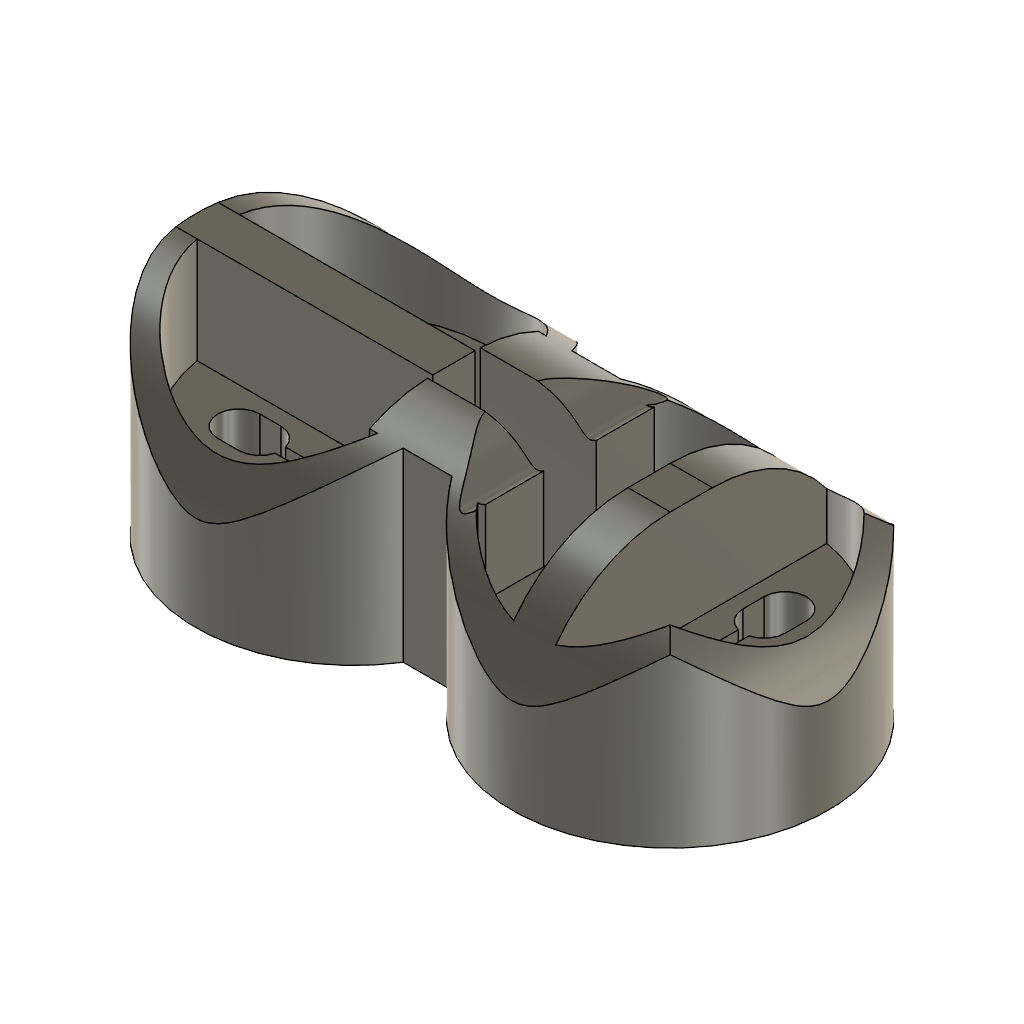
Sensor case Top V1 (Autodesk Fusion 360 design; units mm, degrees)
part number: 2026-09-03-18-15-27-787
Autodesk Fusion 360 part; units mm, degrees
note: some values were not read from the file. Set by a fixed rule: which sketch regions a step uses.
sketch "Sketch1" plane through (0, 0, 0) normal (0, 0, 1) x (1, 0, 0)
  line L0 (1.1557, 4) -> (-1.1557, 4)
  line L1 (1.1557, -4) -> (-1.1557, -4)
  arc A0 (-1.1557, 4) -> (-1.1557, -4) centre (-7.5, 0) ccw
  arc A1 (1.1557, -4) -> (1.1557, 4) centre (7.5, 0) ccw
  line L2 (2.75, 0) -> (-2.75, 0)
  line L3 (0, -1.25) -> (0, 1.25)
  line L4 (-2.75, -1.25) -> (-2.75, 1.25)
  line L5 (2.75, -1.25) -> (2.75, 1.25)
  line L6 (-2.75, 1.25) -> (2.75, 1.25)
  line L7 (2.75, 1.25) -> (2.75, -1.25)
  line L8 (2.75, -1.25) -> (-2.75, -1.25)
  line L9 (-2.75, -1.25) -> (-2.75, 1.25)
  point P0 (0, 4)
  point P1 (0, -4)
  dimension "d1" = 15
  dimension "d2" = 5.5
  dimension "d3" = 2.5
  dimension "d4" = 2.5
  dimension "d5" = 2.5
  constraint coincident origin A0
  constraint coincident origin A1
  constraint midpoint L0 P0
  constraint horizontal L0
  constraint midpoint L1 P1
  constraint horizontal L1
  constraint midpoint L2 origin
  constraint horizontal L2
  constraint midpoint L3 origin
  constraint perpendicular L2 L3
  constraint horizontal L6
  constraint vertical L7
  constraint horizontal L8
  constraint vertical L9
  measures "d1" diameter of A1
  measures "d2" distance of L2.start L2.end
  measures "d3" distance of L3.start L3.end
  measures "d4" distance of L4.start L4.end
  measures "d5" distance of L5.start L5.end
extrude "Extrude1" add sketch "Sketch1" along normal blind 4.5
sketch "Sketch2" plane through (0, 0, 4.5) normal (0, 0, 1) x (-1, 0, 0)
  line L0 (-2.75, 1.25) -> (2.75, 1.25)
  line L1 (2.75, 1.25) -> (2.75, -1.25)
  line L2 (2.75, -1.25) -> (-2.75, -1.25)
  line L3 (-2.75, -1.25) -> (-2.75, 1.25)
  arc A0 (-1.1557, 4) -> (-1.1557, -4) centre (-7.5, 0) ccw
  line L4 (-1.1557, -4) -> (1.1557, -4)
  arc A1 (1.1557, -4) -> (1.1557, 4) centre (7.5, 0) ccw
  line L5 (1.1557, 4) -> (-1.1557, 4)
  line L6 (7.5, 1) -> (7.5, -1)
  line L7 (7.5, -1) -> (7.5, -2.7)
  line L8 (9.25, -2.7) -> (5.75, -2.7)
  line L9 (9.2781, -3.6996) -> (10.2496, -3.7)
  line L10 (9.25, -1.7) -> (10.25, -1.7)
  line L11 (4.75, -3.7) -> (5.75, -3.7)
  line L12 (4.75, -1.7) -> (5.75, -1.7)
  arc A2 (9.25, -1.7) -> (9.2781, -3.6996) centre (9.25, -2.7) ccw
  arc A3 (10.2496, -3.7) -> (10.25, -1.7) centre (10.25, -2.7) ccw
  arc A4 (5.7496, -3.7) -> (5.75, -1.7) centre (5.75, -2.7) ccw
  arc A5 (4.75, -1.7) -> (4.7504, -3.7) centre (4.75, -2.7) ccw
  line L13 (10.25, 1.7) -> (9.25, 1.7)
  arc A6 (9.2504, 3.7) -> (9.25, 1.7) centre (9.25, 2.7) ccw
  line L14 (10.25, 3.7) -> (9.25, 3.7)
  arc A7 (10.25, 1.7) -> (10.2496, 3.7) centre (10.25, 2.7) ccw
  arc A8 (5.75, 1.7) -> (5.7219, 3.6996) centre (5.75, 2.7) ccw
  line L15 (5.7219, 3.6996) -> (4.7504, 3.7)
  line L16 (5.75, 1.7) -> (4.75, 1.7)
  arc A9 (4.7504, 3.7) -> (4.75, 1.7) centre (4.75, 2.7) ccw
  line L17 (5.75, 2.7) -> (9.25, 2.7)
  line L18 (7.5, 1) -> (7.5, 2.7)
  line L19 (7.5, -1) -> (7.5, 1)
  line L20 (-6.5, 0) -> (-8.5, 0)
  line L21 (-8.5, 0) -> (-10.2, 0)
  line L22 (-10.2, -1.75) -> (-10.2, 1.75)
  arc A10 (-9.2, -1.75) -> (-11.1996, -1.7781) centre (-10.2, -1.75) ccw
  line L23 (-9.2, -1.75) -> (-9.2, -2.75)
  arc A11 (-11.2, -2.7496) -> (-9.2, -2.75) centre (-10.2, -2.75) ccw
  line L24 (-11.1996, -1.7781) -> (-11.2, -2.7496)
  line L25 (-11.2, 2.75) -> (-11.2, 1.75)
  arc A12 (-11.2, 1.7504) -> (-9.2, 1.75) centre (-10.2, 1.75) ccw
  arc A13 (-9.2, 2.75) -> (-11.2, 2.7496) centre (-10.2, 2.75) ccw
  line L26 (-9.2, 2.75) -> (-9.2, 1.75)
  line L27 (-6.5, 0) -> (-4.8, 0)
  line L28 (-4.8, 1.75) -> (-4.8, -1.75)
  arc A14 (-5.8, 1.75) -> (-3.8004, 1.7781) centre (-4.8, 1.75) ccw
  line L29 (-5.8, 1.75) -> (-5.8, 2.75)
  arc A15 (-3.8, 2.7496) -> (-5.8, 2.75) centre (-4.8, 2.75) ccw
  line L30 (-3.8004, 1.7781) -> (-3.8, 2.7496)
  line L31 (-3.8, -2.75) -> (-3.8, -1.75)
  arc A16 (-5.8, -2.75) -> (-3.8, -2.7496) centre (-4.8, -2.75) ccw
  line L32 (-5.8, -2.75) -> (-5.8, -1.75)
  arc A17 (-3.8, -1.7504) -> (-5.8, -1.75) centre (-4.8, -1.75) ccw
  point P0 (7.5, 0)
  dimension "d8" = 2
  dimension "d9" = 1.7
  dimension "d10" = 3.5
  dimension "d11" = 2
  dimension "d12" = 2
  dimension "d13" = 2
  dimension "d14" = 2
  dimension "d15" = 2
  dimension "d16" = 1.7
  dimension "d17" = 3.5
  dimension "d18" = 2
  dimension "d19" = 2
  dimension "d20" = 2
  dimension "d21" = 2
  dimension "d22" = 2
  dimension "d23" = 1.7
  dimension "d24" = 3.5
  dimension "d25" = 2
  dimension "d26" = 2
  dimension "d27" = 2
  dimension "d28" = 2
  dimension "d29" = 1.7
  dimension "d30" = 3.5
  dimension "d31" = 2
  dimension "d32" = 2
  dimension "d33" = 2
  dimension "d34" = 2
  constraint midpoint L6 P0
  constraint coincident P0 A1.centre
  constraint vertical L6
  constraint parallel L6 L7
  constraint midpoint L7.end L8
  constraint perpendicular L7 L8
  constraint coincident L8.start A2.centre
  constraint coincident L8.end A4.centre
  constraint coincident L9.end A3
  constraint tangent L9 A3
  constraint tangent L10 A3
  constraint parallel L8 L10
  constraint coincident L9 A3.start
  constraint coincident L11 A5.end
  constraint coincident L11 A4.start
  constraint parallel L18 L19
  constraint midpoint L18.end L17
  constraint perpendicular L17 L18
  constraint coincident A8.centre L17.start
  constraint coincident A6.centre L17.end
  constraint coincident L15.end A9
  constraint tangent L15 A9
  constraint tangent L16 A9
  constraint parallel L16 L17
  constraint coincident A9.start L15
  constraint coincident A7.end L14
  constraint coincident A6.start L14
  constraint parallel L20 L21
  constraint midpoint L21.end L22
  constraint perpendicular L21 L22
  constraint coincident L22.start A10.centre
  constraint coincident L22.end A12.centre
  constraint coincident L24.end A11
  constraint tangent A11 L24
  constraint tangent L23 A11
  constraint parallel L22 L23
  constraint coincident A11.start L24
  constraint coincident A13.end L25
  constraint coincident A12.start L25
  constraint midpoint L27.end L28
  constraint perpendicular L27 L28
  constraint coincident L28.start A14.centre
  constraint coincident L28.end A17.centre
  constraint coincident L30.end A15
  constraint tangent A15 L30
  constraint tangent L29 A15
  constraint parallel L28 L29
  constraint coincident A15.start L30
  constraint coincident A16.end L31
  constraint coincident A17.start L31
  measures "d8" distance of L6.start L6.end
  measures "d9" distance of L6.end L7.end
  measures "d10" distance of L8.start L8.end
  measures "d11" diameter of A2
  measures "d12" diameter of A4
  measures "d13" diameter of A3
  measures "d14" diameter of A5
  measures "d15" distance of L6.end L6.start
  measures "d16" distance of L6.start L18.end
  measures "d17" distance of A8.centre A6.centre
  measures "d18" diameter of A8
  measures "d19" diameter of A6
  measures "d20" diameter of A9
  measures "d21" diameter of A7
  measures "d22" distance of L20.start L20.end
  measures "d23" distance of L20.end L21.end
  measures "d24" distance of L22.start L22.end
  measures "d25" diameter of A10
  measures "d26" diameter of A12
  measures "d27" diameter of A11
  measures "d28" diameter of A13
  measures "d29" distance of L27.end L20.start
  measures "d30" distance of L28.end L28.start
  measures "d31" diameter of A14
  measures "d32" diameter of A17
  measures "d33" diameter of A15
  measures "d34" diameter of A16
extrude "Extrude2" cut sketch "Sketch2" against normal blind 5 contours L9 L10 A2 A3 | L11 L12 A4 A5 | L13 A6 L14 A7 | A8 L15 L16 A9 | A10 L23 A11 L24 | L25 A12 A13 L26 | A14 L29 A15 L30 | L31 A16 L32 A17
sketch "Sketch3" plane through (0, 0, 4.5) normal (0, 0, 1) x (-1, 0, 0)
  arc A0 (-1.1557, 4) -> (-1.1557, -4) centre (-7.5, 0) ccw
  line L0 (-1.1557, -4) -> (1.1557, -4)
  arc A1 (1.1557, -4) -> (1.1557, 4) centre (7.5, 0) ccw
  line L1 (1.1557, 4) -> (-1.1557, 4)
  line L2 (-2.75, 1.25) -> (2.75, 1.25)
  line L3 (2.75, 1.25) -> (2.75, -1.25)
  line L4 (2.75, -1.25) -> (-2.75, -1.25)
  line L5 (-2.75, -1.25) -> (-2.75, 1.25)
  line L6 (-3.8, 2.7496) -> (-3.8004, 1.7781)
  arc A2 (-5.8, 1.75) -> (-3.8004, 1.7781) centre (-4.8, 1.75) ccw
  line L7 (-5.8, 1.75) -> (-5.8, 2.75)
  arc A3 (-3.8, 2.7496) -> (-5.8, 2.75) centre (-4.8, 2.75) ccw
  line L8 (9.25, 3.7) -> (10.2496, 3.7)
  arc A4 (10.25, 1.7) -> (10.2496, 3.7) centre (10.25, 2.7) ccw
  line L9 (10.25, 1.7) -> (9.25, 1.7)
  arc A5 (9.25, 3.7) -> (9.25, 1.7) centre (9.25, 2.7) ccw
  line L10 (10.2496, -3.7) -> (9.2781, -3.6996)
  arc A6 (9.25, -1.7) -> (9.2781, -3.6996) centre (9.25, -2.7) ccw
  line L11 (9.25, -1.7) -> (10.25, -1.7)
  arc A7 (10.2496, -3.7) -> (10.25, -1.7) centre (10.25, -2.7) ccw
  line L12 (-3.8, -1.7504) -> (-3.8, -2.7496)
  arc A8 (-5.8, -2.75) -> (-3.8, -2.7496) centre (-4.8, -2.75) ccw
  line L13 (-5.8, -2.75) -> (-5.8, -1.75)
  arc A9 (-3.8, -1.7504) -> (-5.8, -1.75) centre (-4.8, -1.75) ccw
  arc A10 (-11.2, 1.7504) -> (-9.2, 1.75) centre (-10.2, 1.75) ccw
  line L14 (-11.2, 1.7504) -> (-11.2, 2.7496)
  arc A11 (-9.2, 2.75) -> (-11.2, 2.7496) centre (-10.2, 2.75) ccw
  line L15 (-9.2, 2.75) -> (-9.2, 1.75)
  line L16 (4.7504, 3.7) -> (5.7219, 3.6996)
  arc A12 (5.75, 1.7) -> (5.7219, 3.6996) centre (5.75, 2.7) ccw
  line L17 (5.75, 1.7) -> (4.75, 1.7)
  arc A13 (4.7504, 3.7) -> (4.75, 1.7) centre (4.75, 2.7) ccw
  line L18 (5.7496, -3.7) -> (4.7504, -3.7)
  arc A14 (4.75, -1.7) -> (4.7504, -3.7) centre (4.75, -2.7) ccw
  line L19 (4.75, -1.7) -> (5.75, -1.7)
  arc A15 (5.7496, -3.7) -> (5.75, -1.7) centre (5.75, -2.7) ccw
  line L20 (-11.2, -2.7496) -> (-11.1996, -1.7781)
  arc A16 (-9.2, -1.75) -> (-11.1996, -1.7781) centre (-10.2, -1.75) ccw
  line L21 (-9.2, -1.75) -> (-9.2, -2.75)
  arc A17 (-11.2, -2.7496) -> (-9.2, -2.75) centre (-10.2, -2.75) ccw
  line L22 (7.5, 2.7) -> (7.5, -2.7)
  line L23 (6.7182, -2.45) -> (8.2818, -2.45)
  line L24 (8.2818, -2.45) -> (8.2818, -2.95)
  line L25 (8.2818, -2.95) -> (6.7182, -2.95)
  line L26 (6.7182, -2.95) -> (6.7182, -2.45)
  line L27 (6.7182, -2.45) -> (8.2818, -2.95) construction
  line L28 (8.2818, -2.45) -> (6.7182, -2.95) construction
  line L29 (6.7182, -2.45) -> (8.2818, -2.45)
  line L30 (8.2818, -2.95) -> (6.7182, -2.95)
  line L31 (8.2818, -2.45) -> (8.2818, -2.95)
  line L32 (6.7182, -2.95) -> (6.7182, -2.45)
  line L33 (6.7182, 2.95) -> (8.2818, 2.95)
  line L34 (8.2818, 2.45) -> (6.7182, 2.45)
  line L35 (8.2818, 2.95) -> (8.2818, 2.45)
  line L36 (6.7182, 2.45) -> (6.7182, 2.95)
  line L37 (-10.2, 0) -> (-4.8, 0)
  line L38 (-5.05, -0.7818) -> (-5.05, 0.7818)
  line L39 (-4.55, 0.7818) -> (-4.55, -0.7818)
  line L40 (-5.05, 0.7818) -> (-4.55, 0.7818)
  line L41 (-4.55, -0.7818) -> (-5.05, -0.7818)
  line L42 (-10.45, -0.7818) -> (-10.45, 0.7818)
  line L43 (-9.95, 0.7818) -> (-9.95, -0.7818)
  line L44 (-10.45, 0.7818) -> (-9.95, 0.7818)
  line L45 (-9.95, -0.7818) -> (-10.45, -0.7818)
  point P0 (7.5, 0)
  point P1 (7.5, -2.7)
  point P2 (-7.5, 0)
  dimension "d37" = 5.4
  dimension "d38" = 0.5
  dimension "d39" = 0.5
  dimension "d40" = 0.5
  dimension "d41" = 5.4
  dimension "d42" = 0.5
  dimension "d43" = 0.5
  constraint midpoint L22 P0
  constraint coincident P0 A1.centre
  constraint vertical L22
  constraint horizontal L23
  constraint perpendicular L23 L24
  constraint parallel L23 L25
  constraint parallel L24 L26
  constraint coincident L27 P1
  constraint coincident L28 P1
  constraint coincident A15 L23.start
  constraint coincident P1 L22.end
  constraint horizontal L29
  constraint perpendicular L29 L31
  constraint parallel L29 L30
  constraint parallel L31 L32
  constraint horizontal L33
  constraint perpendicular L33 L35
  constraint parallel L33 L34
  constraint parallel L35 L36
  constraint midpoint L37 P2
  constraint coincident P2 A0.centre
  constraint horizontal L37
  constraint perpendicular L38 L40
  constraint parallel L38 L39
  constraint parallel L40 L41
  constraint perpendicular L42 L44
  constraint parallel L42 L43
  constraint parallel L44 L45
  measures "d37" distance of L22.start P1
  measures "d38" distance of L23.end L24.end
  measures "d39" distance of L23.end L24.end
  measures "d40" distance of L33.end L34.start
  measures "d41" distance of L37.start L37.end
  measures "d42" distance of L38.end L39.start
  measures "d43" distance of L42.end L43.start
extrude "Extrude3" cut sketch "Sketch3" against normal blind 3 contours A2 A9 L38 L39 | A5 A12 L33 L34 | A6 A15 L23 L25 L29 L30 | A10 A16 L42 L43
sketch "Sketch4" plane through (0, 0, 4.5) normal (0, 0, 1) x (-1, 0, 0)
  line L0 (-10.45, -0.7818) -> (-10.45, 0.7818)
  arc A0 (-11.2, 1.7504) -> (-10.45, 0.7818) centre (-10.2, 1.75) ccw
  line L1 (-11.2, 1.7504) -> (-11.2, 2.7496)
  arc A1 (-9.2, 2.75) -> (-11.2, 2.7496) centre (-10.2, 2.75) ccw
  line L2 (-9.2, 2.75) -> (-9.2, 1.75)
  arc A2 (-9.95, 0.7818) -> (-9.2, 1.75) centre (-10.2, 1.75) ccw
  line L3 (-9.95, 0.7818) -> (-9.95, -0.7818)
  arc A3 (-9.2, -1.75) -> (-9.95, -0.7818) centre (-10.2, -1.75) ccw
  line L4 (-9.2, -1.75) -> (-9.2, -2.75)
  arc A4 (-11.2, -2.7496) -> (-9.2, -2.75) centre (-10.2, -2.75) ccw
  line L5 (-11.2, -2.7496) -> (-11.1996, -1.7781)
  arc A5 (-10.45, -0.7818) -> (-11.1996, -1.7781) centre (-10.2, -1.75) ccw
  line L6 (6.7182, -2.45) -> (8.2818, -2.45)
  arc A6 (9.25, -1.7) -> (8.2818, -2.45) centre (9.25, -2.7) ccw
  line L7 (9.25, -1.7) -> (10.25, -1.7)
  arc A7 (10.2496, -3.7) -> (10.25, -1.7) centre (10.25, -2.7) ccw
  line L8 (10.2496, -3.7) -> (9.2781, -3.6996)
  arc A8 (8.2818, -2.95) -> (9.2781, -3.6996) centre (9.25, -2.7) ccw
  line L9 (8.2818, -2.95) -> (6.7182, -2.95)
  arc A9 (5.7496, -3.7) -> (6.7182, -2.95) centre (5.75, -2.7) ccw
  line L10 (5.7496, -3.7) -> (4.7504, -3.7)
  arc A10 (4.75, -1.7) -> (4.7504, -3.7) centre (4.75, -2.7) ccw
  line L11 (4.75, -1.7) -> (5.75, -1.7)
  arc A11 (6.7182, -2.45) -> (5.75, -1.7) centre (5.75, -2.7) ccw
  line L12 (6.7182, 2.95) -> (8.2818, 2.95)
  arc A12 (9.25, 3.7) -> (8.2818, 2.95) centre (9.25, 2.7) ccw
  line L13 (9.25, 3.7) -> (10.2496, 3.7)
  arc A13 (10.25, 1.7) -> (10.2496, 3.7) centre (10.25, 2.7) ccw
  line L14 (10.25, 1.7) -> (9.25, 1.7)
  arc A14 (8.2818, 2.45) -> (9.25, 1.7) centre (9.25, 2.7) ccw
  line L15 (8.2818, 2.45) -> (6.7182, 2.45)
  arc A15 (5.75, 1.7) -> (6.7182, 2.45) centre (5.75, 2.7) ccw
  line L16 (5.75, 1.7) -> (4.75, 1.7)
  arc A16 (4.7504, 3.7) -> (4.75, 1.7) centre (4.75, 2.7) ccw
  line L17 (4.7504, 3.7) -> (5.7219, 3.6996)
  arc A17 (6.7182, 2.95) -> (5.7219, 3.6996) centre (5.75, 2.7) ccw
  line L18 (-5.05, -0.7818) -> (-5.05, 0.7818)
  arc A18 (-5.8, 1.75) -> (-5.05, 0.7818) centre (-4.8, 1.75) ccw
  line L19 (-5.8, 1.75) -> (-5.8, 2.75)
  arc A19 (-3.8, 2.7496) -> (-5.8, 2.75) centre (-4.8, 2.75) ccw
  line L20 (-3.8, 2.7496) -> (-3.8004, 1.7781)
  arc A20 (-4.55, 0.7818) -> (-3.8004, 1.7781) centre (-4.8, 1.75) ccw
  line L21 (-4.55, 0.7818) -> (-4.55, -0.7818)
  arc A21 (-3.8, -1.7504) -> (-4.55, -0.7818) centre (-4.8, -1.75) ccw
  line L22 (-3.8, -1.7504) -> (-3.8, -2.7496)
  arc A22 (-5.8, -2.75) -> (-3.8, -2.7496) centre (-4.8, -2.75) ccw
  line L23 (-5.8, -2.75) -> (-5.8, -1.75)
  arc A23 (-5.05, -0.7818) -> (-5.8, -1.75) centre (-4.8, -1.75) ccw
  line L24 (-2.75, 1.25) -> (2.75, 1.25)
  line L25 (2.75, 1.25) -> (2.75, -1.25)
  line L26 (2.75, -1.25) -> (-2.75, -1.25)
  line L27 (-2.75, -1.25) -> (-2.75, 1.25)
  arc A24 (-1.1557, 4) -> (-1.1557, -4) centre (-7.5, 0) ccw
  line L28 (-1.1557, -4) -> (1.1557, -4)
  arc A25 (1.1557, -4) -> (1.1557, 4) centre (7.5, 0) ccw
  line L29 (1.1557, 4) -> (-1.1557, 4)
  line L30 (2.75, 1) -> (12.25, 1)
  line L31 (12.25, 1) -> (12.25, -1)
  line L32 (12.25, -1) -> (2.75, -1)
  line L33 (2.75, -1) -> (2.75, 1)
  line L34 (2.75, 1) -> (12.25, -1) construction
  line L35 (12.25, 1) -> (2.75, -1) construction
  line L36 (12.25, 1) -> (15, 1)
  line L37 (15, 1) -> (15, -1)
  line L38 (15, -1) -> (12.25, -1)
  line L39 (12.25, -1) -> (12.25, 1)
  line L40 (-6.5, -8) -> (-8.5, -8)
  line L41 (-8.5, -8) -> (-8.5, 8)
  line L42 (-8.5, 8) -> (-6.5, 8)
  line L43 (-6.5, 8) -> (-6.5, -8)
  line L44 (-6.5, -8) -> (-8.5, 8) construction
  line L45 (-8.5, -8) -> (-6.5, 8) construction
  circle A26 centre (-7.5, 0) radius 6.5
  circle A27 centre (-7.5, 0) radius 7.5
  circle A28 centre (-7.5, 0) radius 6.5
  circle A29 centre (-7.5, 0) radius 6.5
  circle A30 centre (7.5, 0) radius 7.5
  circle A31 centre (7.5, 0) radius 6.5
  point P0 (7.5, 0)
  point P1 (-7.5, 0)
  dimension "d46" = 2
  dimension "d47" = 2
  constraint horizontal L30
  constraint perpendicular L30 L31
  constraint parallel L30 L32
  constraint parallel L31 L33
  constraint coincident L34 P0
  constraint coincident L35 P0
  constraint coincident L25 L30.start
  constraint coincident P0 A25.centre
  constraint horizontal L36
  constraint vertical L37
  constraint horizontal L38
  constraint vertical L39
  constraint horizontal L40
  constraint perpendicular L40 L41
  constraint parallel L40 L42
  constraint parallel L41 L43
  constraint coincident L44 P1
  constraint coincident L45 P1
  constraint coincident P1 A24.centre
  constraint concentric A25 A30
  measures "d46" distance of L30.end L31.end
  measures "d47" distance of L40.start L40.end
extrude "Extrude4" add sketch "Sketch4" along normal blind 5 contours L24 A24 L43 A26 A27 A28 A29 | A24 L41 L43 A26 A27 A28 A29 | L41 L43 A26 A28 A29 | L26 A24 L43 A26 A27 A28 A29 | L24 A25 L36 A30 A31 | A24 L41 L43 A26 A27 A28 A29 | A24 L41 A26 A27 A28 A29 | L26 A25 L38 A30 A31 | L31 L36 L38 L39 A31 | A25 L36 L38 A30 A31 | L25 L30 L31 L32 L33 L39
sketch "Sketch8" plane through (0, 0, 4.5) normal (0, 0, 1) x (-1, 0, 0)
  line L0 (1.1557, 4) -> (-1.1557, 4)
  arc A0 (-0.1049, 1.25) -> (-1.1557, 4) centre (-7.5, 0) ccw
  line L1 (-0.1049, 1.25) -> (0.1049, 1.25)
  arc A1 (1.1557, 4) -> (0.1049, 1.25) centre (7.5, 0) ccw
  line L2 (0, -4) -> (3, -4)
  line L3 (2.75, -1.25) -> (2.75, -4)
  line L4 (0, 4) -> (-3, 4)
  line L5 (-2.75, 1.25) -> (-2.75, 4)
  line L6 (2.75, -4) -> (-2.75, -4)
  line L7 (-2.75, -4) -> (-2.75, 4)
  line L8 (-2.75, 4) -> (2.75, 4)
  line L9 (2.75, 4) -> (2.75, -4)
  line L10 (2.75, -1.25) -> (-2.75, -1.25)
  line L11 (-2.75, -1.25) -> (-2.75, 1.25)
  line L12 (-2.75, 1.25) -> (2.75, 1.25)
  line L13 (2.75, 1.25) -> (2.75, -1.25)
  constraint horizontal L2
  constraint coincident L2 L3.end
  constraint perpendicular L2 L3
  constraint midpoint L0 L4.start
  constraint perpendicular L3 L4
  constraint coincident L4 L5.end
  constraint perpendicular L4 L5
  constraint horizontal L6
  constraint vertical L7
  constraint horizontal L8
  constraint vertical L9
  constraint horizontal L10
  constraint vertical L11
  constraint horizontal L12
  constraint vertical L13
extrude "Extrude8" add sketch "Sketch8" along normal blind 5 contours L0 A0 L1 A1 L4 L8 L12 | A1 L8 L9 L12 | A0 L4 L5 L7 L8 L12 | L2 L3 L6 L7 L9 L10
sketch "Sketch5" plane through (-2.75, 0, 0) normal (1, 0, 0) x (0, 1, 0)
  line L0 (-1.25, 0) -> (1.25, 0)
  line L1 (1.25, 0) -> (1.25, 4.5)
  line L2 (1.25, 4.5) -> (1, 4.5)
  line L3 (1, 4.5) -> (1, 9.5)
  line L4 (1, 9.5) -> (-1, 9.5)
  line L5 (-1, 9.5) -> (-1, 4.5)
  line L6 (-1.25, 4.5) -> (-1.25, 0)
  line L7 (1, 9.5) -> (-1, 9.5)
  line L8 (-1, 9.5) -> (-1, 0.5)
  line L9 (-1, 0.5) -> (1, 0.5)
  line L10 (1, 0.5) -> (1, 9.5)
  line L11 (1, 9.5) -> (-1, 0.5) construction
  line L12 (-1, 9.5) -> (1, 0.5) construction
  line L13 (0, 9.5) -> (0, 4.5)
  line L14 (7.5, 4.5) -> (-7.5, 4.5)
  arc A0 (7.5, 4.5) -> (1, 9.5) centre (1, 2.775) ccw
  arc A1 (-1, 9.5) -> (-7.5, 4.5) centre (-1, 2.775) ccw
  line L15 (7.5, 9.5) -> (-7.5, 9.5)
  line L16 (-7.5, 9.5) -> (-7.5, 4.5)
  line L17 (-7.5, 4.5) -> (7.5, 4.5)
  line L18 (7.5, 4.5) -> (7.5, 9.5)
  line L19 (-1, 4.5) -> (-1.25, 4.5)
  point P0 (0, 5)
  dimension "d50" = 5
  constraint horizontal L7
  constraint perpendicular L7 L8
  constraint parallel L7 L9
  constraint parallel L8 L10
  constraint coincident L11 P0
  constraint coincident L12 P0
  constraint coincident L3.end L4.start
  constraint midpoint L7 L13.start
  constraint perpendicular L7 L13
  constraint midpoint L13.end L14
  constraint perpendicular L13 L14
  constraint tangent L4 A0
  constraint tangent L7 A1
  constraint horizontal L15
  constraint vertical L16
  constraint horizontal L17
  constraint vertical L18
  measures "d50" distance of L13.start L13.end
extrude "Extrude5" cut sketch "Sketch5" along normal blind 18.5 and the other way blind 13 contours A1 L15 L16 | A0 L15 L18
sketch "Sketch6" plane through (0, -1.25, 0) normal (0, 1, 0) x (-1, 0, 0)
  line L0 (2.75, 9.4954) -> (-2.75, 9.4954)
  line L1 (-2.75, 4.5) -> (-2.75, 0)
  line L2 (-2.75, 0) -> (2.75, 0)
  line L3 (2.75, 0) -> (2.75, 4.5)
  line L4 (-6.5, 9.5, 2.25) -> (-6.5, 9.5, 0.25)
  line L5 (-8.5, 9.5, 0.25) -> (-8.5, 9.5, 2.25)
  line L6 (-6.5, 9.5) -> (-8.5, 9.5)
  line L7 (-7.5, 9.5) -> (-7.5, 0)
  line L8 (-7.5, 9.5) -> (-7.5, 4.5)
  line L9 (-15, 4.5) -> (0, 4.5)
  arc A0 (-0.1049, 4.5) -> (-6.5, 9.5) centre (-6.25, 3.23) ccw
  arc A1 (-8.5, 9.5) -> (-15, 4.5) centre (-8.5, 2.775) ccw
  line L10 (0.05, 9.5) -> (-15, 9.5)
  line L11 (-15, 9.5) -> (-15, 4.5)
  line L12 (-15, 4.5) -> (0.05, 4.5)
  line L13 (0.05, 4.5) -> (0.05, 9.5)
  line L14 (-2.75, 9.4954) -> (-2.75, 4.5)
  line L15 (2.75, 4.5) -> (2.75, 9.4954)
  spline S0 degree 5 poles (-6.5, 9.5) (-6.2948, 9.5232) (-5.8956, 9.5547) (-5.3307, 9.5574) (-4.6467, 9.4712) (-3.9122, 9.2176) (-3.3052, 8.8572) (-2.8231, 8.4666) (-2.4597, 8.2331) (-2.1651, 8.373) (-1.7833, 8.7735) (-1.267, 9.1481) (-0.6906, 9.3623) (-0.2125, 9.4614) (0.05, 9.5) knots 0 0 0 0 0 0 0.1 0.2 0.3 0.4 0.5 0.6 0.7 0.8 0.9 1 1 1 1 1 1
  line L16 (-3.1084, 8.6619) -> (-2.3916, 8.2145)
  line L17 (-1.35, 9.2941) -> (1.45, 9.7059)
  point P0 (-2.75, 8.4382)
  dimension "d56" = 2
  dimension "d57" = 5
  dimension "d58" = 15
  constraint midpoint L6 L7.start
  constraint perpendicular L6 L7
  constraint perpendicular L6 L8
  constraint midpoint L8.end L9
  constraint perpendicular L8 L9
  constraint horizontal L10
  constraint vertical L11
  constraint horizontal L12
  constraint vertical L13
  constraint coincident L14 P0
  constraint coincident A0 P0
  constraint midpoint P0 L16
  constraint coincident A0 L16.start
  constraint midpoint L10.start L17
  measures "d56" distance of L6.start L6.end
  measures "d57" distance of L7.start L8.end
  measures "d58" distance of L9.start L9.end
extrude "Extrude6" cut sketch "Sketch6" along normal blind 9 and the other way blind 7 contours L0 L10 L14 S0 | A0 L10 L14 S0 L16 | A0 L10 S0 | A1 L10 L11
